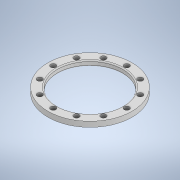
# Autodesk Inventor part: top ring
Saved by Autodesk Inventor 2021 (Build 250183000, 183)
## iProperties
Created: 2022-10-28
Part Number: top ring
Material: Generic
Document SubType Name: Modeling
Designer: warre
Density: 1 g/cm^3
Appearance: Default
Author: warre
Autodesk Inventor part; units mm, degrees
ref_plane "YZ Plane" through (0, 0, 0) normal (1, 0, 0) x (0, 1, 0)
ref_plane "XZ Plane" through (0, 0, 0) normal (0, 1, 0) x (-1, 0, 0)
ref_plane "XY Plane" through (0, 0, 0) normal (0, 0, 1) x (1, 0, 0)
sketch "Sketch1" plane through (0, 0, 0) normal (0, 1, 0) x (-1, 0, 0)
  circle A0 centre (0, 0) radius 31
  circle A1 centre (0, 0) radius 40
  circle A2 centre (0, 0) radius 35 construction
  circle A3 centre (35, 0) radius 2.5
  circle A4 centre (30.3109, 17.5) radius 2.5
  circle A5 centre (17.5, 30.3109) radius 2.5
  circle A6 centre (0, 35) radius 2.5
  circle A7 centre (-17.5, 30.3109) radius 2.5
  circle A8 centre (-30.3109, 17.5) radius 2.5
  circle A9 centre (-35, 0) radius 2.5
  circle A10 centre (-30.3109, -17.5) radius 2.5
  circle A11 centre (-17.5, -30.3109) radius 2.5
  circle A12 centre (0, -35) radius 2.5
  circle A13 centre (17.5, -30.3109) radius 2.5
  circle A14 centre (30.3109, -17.5) radius 2.5
  dimension "d2" = 70
  dimension "d0" = 62
  dimension "d1" = 80
  dimension "d3" = 5
  dimension "d6" = 360
  constraints: 14 centre point, 3 coincident, 1 horizontal alignment, 27 other
  measures "d0" diameter of A0
  measures "d1" diameter of A1
  measures "d3" diameter of A3
extrude "Extrusion1" add sketch "Sketch1" along normal blind 5
fillet "Fillet1" radius 1 2 edges at (31, 0, 0) (31, 5, 0)
body "Solid1"
